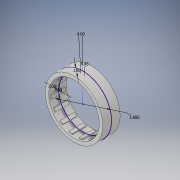
# Autodesk Inventor part: Eh
Saved by Autodesk Inventor 2017 (Build 210142000, 142)
## iProperties
Created: 2020-02-27
Part Number: Eh
Material: Generic
Document SubType Name: Modeling
Designer: 10042265
Density: 1 g/cm^3
Appearance: Default
Author: 10042265
Autodesk Inventor part; units mm, degrees
ref_plane "YZ Plane" through (0, 0, 0) normal (1, 0, 0) x (0, 1, 0)
ref_plane "XZ Plane" through (0, 0, 0) normal (0, 1, 0) x (-1, 0, 0)
ref_plane "XY Plane" through (0, 0, 0) normal (0, 0, 1) x (1, 0, 0)
sketch "Sketch1" plane through (0, 0, 0) normal (0, 0, 1) x (1, 0, 0)
  circle A0 centre (0, 0) radius 20.955
  circle A1 centre (0, 0) radius 18.415
  line L0 (-1.2314, 17.61) -> (-1.2846, 18.3701)
  line L1 (1.2314, 17.61) -> (1.2846, 18.3701)
  line L2 (0, 0) -> (0, 24.6774) construction
  arc A2 (1.2314, 17.61) -> (-1.2314, 17.61) centre (0, 0) ccw
  circle A3 centre (0, 0) radius 17.653
  dimension "d0" = 41.91
  dimension "d1" = 2.54
  dimension "d4" = 4
  dimension "d5" = 4
  dimension "d7" = 0.762
  dimension "d13" = 0.762
  constraints: 6 end point, 4 centre point, 4 point on circle, 2 coincident, 1 vertical
  measures "d0" diameter of A0
  measures "d1" radial gap between concentric circles of A1 A0
  measures "d4" angle of L0 L2
  measures "d5" angle of L2 L1
  measures "d7" radial gap between concentric circles of A1 A2
  measures "d13" radial gap between concentric circles of A1 A3
extrude "Extrusion1" add sketch "Sketch1" along normal mid plane 12.7
extrude "Extrusion2" add sketch "Sketch1" along normal mid plane 10.16 contours L1 A2 L0 A1
pattern_circular "Circular Pattern1" count 15 over 360 about axis through (0, 0, 0) along (0, 0, 1) of "Extrusion2"
extrude "Extrusion3" add sketch "Sketch1" along normal mid plane 1.27 contours A1 L0 A3 L1
body "Solid1"
